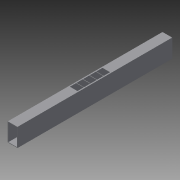
# Autodesk Inventor part: Waveguide
Saved by Autodesk Inventor 2014 (Build 180170000, 170)
## iProperties
Created: 2014-05-15
Part Number: Waveguide
Material: Generic
Document SubType Name: Modeling
Designer: ijs09
Density: 1 g/cm^3
Appearance: Default
Author: ijs09
Autodesk Inventor part; units mm, degrees
ref_plane "YZ Plane" through (0, 0, 0) normal (1, 0, 0) x (0, 1, 0)
ref_plane "XZ Plane" through (0, 0, 0) normal (0, 1, 0) x (-1, 0, 0)
ref_plane "XY Plane" through (0, 0, 0) normal (0, 0, 1) x (1, 0, 0)
sketch "Sketch1" plane through (0, 0, 0) normal (0, 1, 0) x (-1, 0, 0)
  line L0 (3.9497, -7.8994) -> (-3.9497, -7.8994)
  line L1 (-3.9497, -7.8994) -> (-3.9497, 7.8994)
  line L2 (-3.9497, 7.8994) -> (3.9497, 7.8994)
  line L3 (3.9497, 7.8994) -> (3.9497, -7.8994)
  line L4 (4.4497, -8.3994) -> (-4.4497, -8.3994)
  line L5 (-4.4497, -8.3994) -> (-4.4497, 8.3994)
  line L6 (-4.4497, 8.3994) -> (4.4497, 8.3994)
  line L7 (4.4497, 8.3994) -> (4.4497, -8.3994)
  point P0 (0, 0)
  dimension "d0" = 15.7988
  dimension "d1" = 16.7988
  dimension "d2" = 7.8994
  dimension "d3" = 8.3994
  dimension "d4" = 7.8994
  dimension "d5" = 3.9497
  dimension "d6" = 8.8994
  dimension "d7" = 4.4497
  constraints: 16 end point, 4 parallel, 2 horizontal, 2 perpendicular
  measures "d0" distance between parallel lines of L0 L2
  measures "d1" distance between parallel lines of L4 L6
  measures "d2" distance from line of point (0, 0) L0
  measures "d3" distance from line of point (0, 0) L4
  measures "d4" distance between parallel lines of L1 L3
  measures "d5" distance from line of point (0, 0) L1
  measures "d6" distance between parallel lines of L7 L5
  measures "d7" distance from line of point (0, 0) L5
extrude "Extrusion1" add sketch "Sketch1" against normal blind 142
sketch "Sketch2" plane through (4.4497, 0, -8.3994) normal (0, 0, -1) x (-1, 0, 0)
  line L0 (8.8994, 0) -> (0, 0) projected
  line L1 (0, 0) -> (0, -142) projected
  line L2 (8.8994, 0) -> (8.8994, -142) projected
  line L3 (-7.7677, -71) -> (26.0331, -71) construction
  line L4 (7.8994, -73.9) -> (1, -73.9)
  line L5 (1, -73.9) -> (1, -68.1)
  line L6 (1, -68.1) -> (7.8994, -68.1)
  line L7 (7.8994, -68.1) -> (7.8994, -73.9)
  line L8 (7.8994, -67.85) -> (1, -67.85)
  line L9 (1, -67.85) -> (1, -62.05)
  line L10 (1, -62.05) -> (7.8994, -62.05)
  line L11 (7.8994, -62.05) -> (7.8994, -67.85)
  line L12 (7.8994, -61.8) -> (1, -61.8)
  line L13 (1, -61.8) -> (1, -56)
  line L14 (1, -56) -> (7.8994, -56)
  line L15 (7.8994, -56) -> (7.8994, -61.8)
  line L16 (7.8994, -74.15) -> (1, -74.15)
  line L17 (1, -74.15) -> (1, -79.95)
  line L18 (1, -79.95) -> (7.8994, -79.95)
  line L19 (7.8994, -79.95) -> (7.8994, -74.15)
  line L20 (7.8994, -80.2) -> (1, -80.2)
  line L21 (1, -80.2) -> (1, -86)
  line L22 (1, -86) -> (7.8994, -86)
  line L23 (7.8994, -86) -> (7.8994, -80.2)
  point P0 (4.4497, 0)
  dimension "d12" = 71
  dimension "d13" = 5.8
  dimension "d14" = 2.9
  dimension "d15" = 5.8
  dimension "d16" = 5.8
  dimension "d17" = 0.25
  dimension "d18" = 0.25
  dimension "d19" = 5.8
  dimension "d20" = 5.8
  dimension "d25" = 0.25
  dimension "d26" = 0.25
  dimension "d27" = 1
  dimension "d28" = 1
  dimension "d29" = 1
  dimension "d30" = 1
  dimension "d31" = 1
  dimension "d32" = 1
  dimension "d33" = 1
  dimension "d34" = 1
  dimension "d35" = 1
  dimension "d36" = 1
  constraints: 42 end point, 10 parallel, 5 horizontal, 5 perpendicular
  measures "d12" distance between parallel lines of L0 L3
  measures "d13" distance between parallel lines of L6 L4
  measures "d14" distance between parallel lines of L6 L3
  measures "d15" distance between parallel lines of L10 L8
  measures "d16" distance between parallel lines of L14 L12
  measures "d17" distance between parallel lines of L8 L6
  measures "d18" distance between parallel lines of L12 L10
  measures "d19" distance between parallel lines of L18 L16
  measures "d20" distance between parallel lines of L20 L22
  measures "d25" distance between parallel lines of L4 L16
  measures "d26" distance between parallel lines of L18 L20
  measures "d27" distance between parallel lines of L15 L2
  measures "d28" distance between parallel lines of L11 L2
  measures "d29" distance between parallel lines of L7 L2
  measures "d30" distance between parallel lines of L19 L2
  measures "d31" distance between parallel lines of L23 L2
  measures "d32" distance between parallel lines of L1 L21
  measures "d33" distance between parallel lines of L1 L17
  measures "d34" distance between parallel lines of L1 L5
  measures "d35" distance between parallel lines of L1 L9
  measures "d36" distance between parallel lines of L1 L13
extrude "Extrusion2" cut sketch "Sketch2" against normal through all
equation "\"d2\" = 0.5 * d0"
equation "\"d3\" = 0.5 * d1"
equation "\"d5\" = 0.5 * d4"
equation "\"d7\" = 0.5 * d6"
equation "\"d14\" = 0.5 * d13"
equation "\"d15\" = d13"
equation "\"d16\" = d13"
equation "\"d19\" = d13"
equation "\"d20\" = d13"
equation "\"d28\" = d27"
equation "\"d29\" = d27"
equation "\"d30\" = d27"
equation "\"d31\" = d27"
equation "\"d32\" = d27"
equation "\"d33\" = d27"
equation "\"d34\" = d27"
equation "\"d35\" = d27"
equation "\"d36\" = d27"
body "Solid1"
